Autodesk Inventor part; units mm, degrees
(part 2 of 2)
  line L117 (6.1961, 43.2003) -> (8.3839, 43.2003)
  point P0 (0, 0)
  constraints: 2 other
extrude "Extrusion16" cut sketch "Sketch15" against normal blind 4
body "Solid1"
